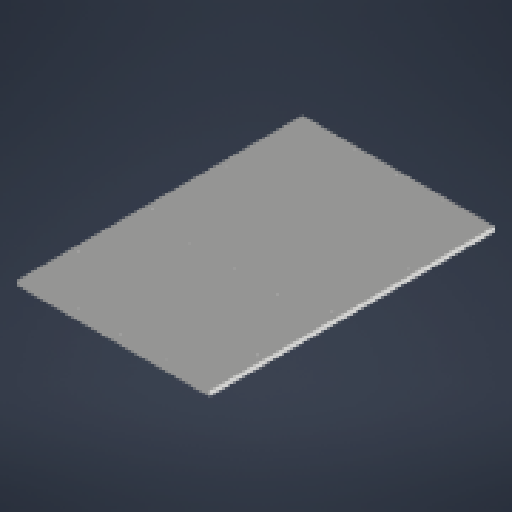
# Autodesk Inventor part: TeflonPlate
Saved by Autodesk Inventor 2027 (Build 310192060, 192F)
## iProperties
Created: 2026-06-12
Part Number: TeflonPlate
Material: Generic
Document SubType Name: Modeling
Designer: kw
Density: 1 g/cm^3
Appearance: Default
Author: kw
Autodesk Inventor part; units mm, degrees
ref_plane "YZ Plane" through (0, 0, 0) normal (1, 0, 0) x (0, 1, 0)
ref_plane "XZ Plane" through (0, 0, 0) normal (0, 1, 0) x (-1, 0, 0)
ref_plane "XY Plane" through (0, 0, 0) normal (0, 0, 1) x (1, 0, 0)
sketch "Sketch1" plane through (0, 0, 0) normal (0, 1, 0) x (-1, 0, 0)
  line L0 (-10, 0) -> (-310, 0)
  line L1 (-310, 0) -> (-310, -500)
  line L2 (-310, -500) -> (-10, -500)
  line L3 (-10, -500) -> (-10, 0)
  line L4 (-310, -500) -> (-320, -500)
  line L5 (-320, -500) -> (-320, 0)
  line L6 (-320, 0) -> (-310, 0)
  line L7 (-310, 0) -> (-310, -500)
  line L8 (-320, -460) -> (-10, -460)
  dimension "d101" = 300
  dimension "d102" = 500
  dimension "d110" = 10
  constraints: 18 end point, 4 parallel, 3 perpendicular, 2 horizontal, 2 point on line
  measures "d101" distance of L2.end L1.end
  measures "d102" distance of L1.end L0.end
  measures "d110" distance of L5.end L6.end
extrude "Extrusion1" add sketch "Sketch1" along normal blind 8 contours L3 L8 L1 L0 | L1 L8 L5 L6
sketch "Sketch5" plane through (0, 8, 0) normal (0, 1, 0) x (1, 0, 0)
  line L0 (10, 0) -> (10, 130)
  line L1 (0, 0) -> (320, 0) projected
  line L2 (10, 0) -> (140, 0) construction
  line L3 (10, 130) -> (10, 250)
  line L4 (10, 250) -> (10, 370)
  line L5 (10, 370) -> (10, 500)
  point P0 (310, 370)
  point P1 (310, 250)
  point P2 (310, 130)
  point P3 (20, 370)
  point P4 (20, 250)
  point P5 (20, 130)
  dimension "d111" = 130
  dimension "d112" = 90
  dimension "d113" = 120
  dimension "d114" = 120
  dimension "d115" = 130
  constraints: 10 end point, 3 point on line, 2 perpendicular, 1 horizontal
  measures "d111" distance of L0.start L0.end
  measures "d112" angle of L2 L0
  measures "d113" distance of L0.end L3.end
  measures "d114" distance of L3.end L4.end
  measures "d115" distance of L4.end L5.end
hole "Hole2" at (310, 8, -130) at (310, 8, -250) at (310, 8, -370) at (20, 8, -130) at (20, 8, -250) at (20, 8, -370) direction (0, -1, 0) diameter 4.3 end through all clearance for "Socket Head Cap Screw ISO 4762" size "M4" standard "ISO"
sketch "Sketch6" plane through (0, 8, 0) normal (0, 1, 0) x (1, 0, 0)
  line L0 (10, 460) -> (10, 0) projected
  line L1 (10, 5) -> (320, 5)
  line L2 (320, 0) -> (320, 460) projected
  line L3 (10, 5) -> (20, 5)
  line L4 (20, 5) -> (100, 5)
  line L5 (100, 5) -> (170, 5)
  line L6 (170, 5) -> (240, 5)
  line L7 (240, 5) -> (320, 5)
  point P0 (0, 0)
  point P1 (10, 500)
  point P2 (320, 500)
  dimension "d143" = 10
  dimension "d144" = 80
  dimension "d145" = 70
  dimension "d146" = 70
  constraints: 12 end point, 5 point on line, 1 collinear, 1 horizontal, 1 other
  measures "d143" distance of L1.start L3.end
  measures "d144" distance of L3.end L4.end
  measures "d145" distance of L4.end L5.end
  measures "d146" distance of L5.end L6.end
hole "Hole3" at (100, 8, -5) at (170, 8, -5) at (240, 8, -5) direction (0, -1, 0) diameter 3.4 end through all clearance for "Socket Head Cap Screw ISO 4762" size "M3" standard "ISO"
sketch "Sketch7" plane through (0, 0, 0) normal (0, -1, 0) x (1, 0, 0)
  line L0 (10, -260) -> (320, -260)
  line L1 (320, 0) -> (320, -460) projected
  line L2 (10, -260) -> (320, -260) construction
  point P0 (0, 0)
  point P1 (320, -500)
  point P2 (100, -270)
  point P3 (170, -270)
  point P4 (240, -270)
  point P5 (100, -450)
  point P6 (170, -450)
  point P7 (240, -450)
  dimension "d148" = 0
  dimension "d151" = 180
  constraints: 4 end point, 1 collinear, 1 horizontal, 1 point on line, 1 vertical, 3 other
  measures "d148" distance between parallel lines of L0 L2
  measures "d151" distance of point (100, -270) point (100, -450)
hole "Hole4" at (100, 0, -270) at (170, 0, -270) at (240, 0, -270) at (100, 0, -450) at (170, 0, -450) at (240, 0, -450) direction (0, 1, 0) diameter 3.4 end through all clearance for "Socket Head Cap Screw ISO 4762" size "M3" standard "ISO"
body "Solid1"
